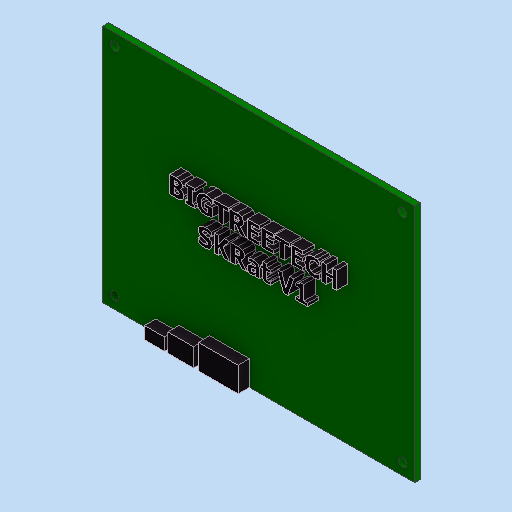
# Autodesk Inventor part: Bigtreetech Skrat V1
Saved by Autodesk Inventor 2023.2 (Build 272271000, 271)
## iProperties
Created: 2024-02-13
Part Number: Bigtreetech Skrat V1
Material: Generisch
Document SubType Name: Modeling
Designer: Nils Bade
Density: 1 g/cm^3
Appearance: Vorgabe
Auf Bestellliste: True
Author: Nils Bade
Autodesk Inventor part; units mm, degrees
ref_plane "YZ Plane" through (0, 0, 0) normal (1, 0, 0) x (0, 1, 0)
ref_plane "XZ Plane" through (0, 0, 0) normal (0, 1, 0) x (-1, 0, 0)
ref_plane "XY Plane" through (0, 0, 0) normal (0, 0, 1) x (1, 0, 0)
sketch "Skizze1" plane through (0, 0, 0) normal (0, 0, 1) x (1, 0, 0)
  line L0 (0, 0) -> (109.67, 0)
  line L1 (109.67, 0) -> (109.67, 84.3)
  line L2 (109.67, 84.3) -> (0, 84.3)
  line L3 (0, 84.3) -> (0, 0)
  circle A0 centre (3.98, 4) radius 1.5
  circle A1 centre (3.98, 80.1) radius 1.5
  circle A2 centre (105.33, 4) radius 1.5
  circle A3 centre (105.33, 80.1) radius 1.5
  line L4 (18.6, 0) -> (25.6, 0)
  line L5 (25.6, 0) -> (25.6, 4.3544)
  line L6 (25.6, 4.3544) -> (18.6, 4.3544)
  line L7 (18.6, 4.3544) -> (18.6, 0)
  line L8 (26.81, 0) -> (35.81, 0)
  line L9 (35.81, 0) -> (35.81, 6.5)
  line L10 (35.81, 6.5) -> (26.81, 6.5)
  line L11 (26.81, 6.5) -> (26.81, 0)
  line L12 (51.54, 0) -> (37.54, 0)
  line L13 (37.54, 0) -> (37.54, 8.7146)
  line L14 (37.54, 8.7146) -> (51.54, 8.7146)
  line L15 (51.54, 8.7146) -> (51.54, 0)
  line L16 (14.8977, 55.016) -> (98.7322, 55.016) construction
  line L17 (98.7322, 55.016) -> (98.7322, 43.3287) construction
  line L18 (98.7322, 43.3287) -> (14.8977, 43.3287) construction
  line L19 (14.8977, 43.3287) -> (14.8977, 55.016) construction
  circle A4 centre (3.98, 4) radius 3.5
  circle A5 centre (3.98, 80.1) radius 3.5
  circle A6 centre (105.33, 80.1) radius 3.5
  circle A7 centre (105.33, 4) radius 3.5
  spline S0 degree 2 poles (32.3655, 50.6659) (32.3655, 50.2112) (32.0194, 49.524) (31.7327, 49.2966) knots 0 0 0 1 2 2 2
  spline S1 degree 2 poles (31.7327, 49.2966) (31.3867, 49.0248) (30.5661, 48.7974) (29.9284, 48.7974) knots 0 0 0 1 2 2 2
  line L20 (29.9284, 48.7974) -> (27.4914, 48.7974)
  line L21 (27.4914, 48.7974) -> (27.4914, 54.8974)
  line L22 (27.4914, 54.8974) -> (29.6417, 54.8974)
  spline S2 degree 2 poles (29.6417, 54.8974) (30.314, 54.8974) (31.0061, 54.7936) (31.3076, 54.6304) knots 0 0 0 1 2 2 2
  spline S3 degree 2 poles (31.3076, 54.6304) (31.6388, 54.4574) (31.9601, 53.8642) (31.9601, 53.4787) knots 0 0 0 1 2 2 2
  spline S4 degree 2 poles (31.9601, 53.4787) (31.9601, 53.0338) (31.5152, 52.3368) (31.1198, 52.1736) knots 0 0 0 1 2 2 2
  line L23 (31.1198, 52.1736) -> (31.1198, 52.144)
  spline S5 degree 2 poles (31.1198, 52.144) (31.6882, 52.0253) (32.3655, 51.2888) (32.3655, 50.6659) knots 0 0 0 1 2 2 2
  spline S6 degree 2 poles (30.7836, 50.6907) (30.7836, 50.9774) (30.5562, 51.2987) (30.3288, 51.3827) knots 0 0 0 1 2 2 2
  spline S7 degree 2 poles (30.3288, 51.3827) (30.1904, 51.4371) (29.701, 51.447) (29.2957, 51.447) knots 0 0 0 1 2 2 2
  line L24 (29.2957, 51.447) -> (29.0139, 51.447)
  line L25 (29.0139, 51.447) -> (29.0139, 49.9096)
  line L26 (29.0139, 49.9096) -> (29.098, 49.9096)
  spline S8 degree 2 poles (29.098, 49.9096) (29.6912, 49.9096) (30.1459, 49.9244) (30.3832, 50.0283) knots 0 0 0 1 2 2 2
  spline S9 degree 2 poles (30.3832, 50.0283) (30.5908, 50.1222) (30.7836, 50.4682) (30.7836, 50.6907) knots 0 0 0 1 2 2 2
  spline S10 degree 2 poles (30.403, 53.1771) (30.403, 53.3254) (30.2498, 53.6368) (30.0916, 53.7061) knots 0 0 0 1 2 2 2
  spline S11 degree 2 poles (30.0916, 53.7061) (29.9433, 53.7753) (29.528, 53.7851) (29.1177, 53.7851) knots 0 0 0 1 2 2 2
  line L27 (29.1177, 53.7851) -> (29.0139, 53.7851)
  line L28 (29.0139, 53.7851) -> (29.0139, 52.49)
  line L29 (29.0139, 52.49) -> (29.2067, 52.49)
  spline S12 degree 2 poles (29.2067, 52.49) (29.5972, 52.49) (29.9136, 52.5048) (30.0817, 52.5839) knots 0 0 0 1 2 2 2
  spline S13 degree 2 poles (30.0817, 52.5839) (30.2646, 52.6729) (30.403, 52.9744) (30.403, 53.1771) knots 0 0 0 1 2 2 2
  line L30 (36.2805, 48.7974) -> (32.9982, 48.7974)
  line L31 (32.9982, 48.7974) -> (32.9982, 49.8602)
  line L32 (32.9982, 49.8602) -> (33.8732, 49.8602)
  line L33 (33.8732, 49.8602) -> (33.8732, 53.8346)
  line L34 (33.8732, 53.8346) -> (32.9982, 53.8346)
  line L35 (32.9982, 53.8346) -> (32.9982, 54.8974)
  line L36 (32.9982, 54.8974) -> (36.2805, 54.8974)
  line L37 (36.2805, 54.8974) -> (36.2805, 53.8346)
  line L38 (36.2805, 53.8346) -> (35.4056, 53.8346)
  line L39 (35.4056, 53.8346) -> (35.4056, 49.8602)
  line L40 (35.4056, 49.8602) -> (36.2805, 49.8602)
  line L41 (36.2805, 49.8602) -> (36.2805, 48.7974)
  spline S14 degree 2 poles (42.3904, 49.1434) (41.99, 48.9803) (40.7097, 48.6689) (40.0869, 48.6689) knots 0 0 0 1 2 2 2
  spline S15 degree 2 poles (40.0869, 48.6689) (38.6484, 48.6689) (36.9429, 50.3298) (36.9429, 51.8523) knots 0 0 0 1 2 2 2
  spline S16 degree 2 poles (36.9429, 51.8523) (36.9429, 53.2859) (38.6484, 55.016) (40.1314, 55.016) knots 0 0 0 1 2 2 2
  spline S17 degree 2 poles (40.1314, 55.016) (40.8976, 55.016) (41.8566, 54.7244) (42.3657, 54.4772) knots 0 0 0 1 2 2 2
  line L42 (42.3657, 54.4772) -> (42.3657, 53.0437)
  line L43 (42.3657, 53.0437) -> (42.2273, 53.0437)
  spline S18 degree 2 poles (42.2273, 53.0437) (42.1186, 53.1277) (41.7033, 53.449) (41.5056, 53.5578) knots 0 0 0 1 2 2 2
  spline S19 degree 2 poles (41.5056, 53.5578) (41.2782, 53.6912) (40.6751, 53.8791) (40.339, 53.8791) knots 0 0 0 1 2 2 2
  spline S20 degree 2 poles (40.339, 53.8791) (39.9485, 53.8791) (39.3009, 53.6319) (39.0488, 53.3798) knots 0 0 0 1 2 2 2
  spline S21 degree 2 poles (39.0488, 53.3798) (38.8066, 53.1326) (38.5248, 52.3763) (38.5248, 51.877) knots 0 0 0 1 2 2 2
  spline S22 degree 2 poles (38.5248, 51.877) (38.5248, 50.8093) (39.5975, 49.791) (40.5219, 49.791) knots 0 0 0 1 2 2 2
  spline S23 degree 2 poles (40.5219, 49.791) (40.6059, 49.791) (40.8234, 49.8009) (40.9075, 49.8058) knots 0 0 0 1 2 2 2
  line L44 (40.9075, 49.8058) -> (40.9075, 51.007)
  line L45 (40.9075, 51.007) -> (39.726, 51.007)
  line L46 (39.726, 51.007) -> (39.726, 52.1489)
  line L47 (39.726, 52.1489) -> (42.3904, 52.1489)
  line L48 (42.3904, 52.1489) -> (42.3904, 49.1434)
  line L49 (44.7187, 48.7974) -> (44.7187, 53.7357)
  line L50 (44.7187, 53.7357) -> (42.9144, 53.7357)
  line L51 (42.9144, 53.7357) -> (42.9144, 54.8974)
  line L52 (42.9144, 54.8974) -> (48.0554, 54.8974)
  line L53 (48.0554, 54.8974) -> (48.0554, 53.7357)
  line L54 (48.0554, 53.7357) -> (46.2511, 53.7357)
  line L55 (46.2511, 53.7357) -> (46.2511, 48.7974)
  line L56 (46.2511, 48.7974) -> (44.7187, 48.7974)
  line L57 (54.3186, 48.7974) -> (52.4549, 48.7974)
  line L58 (52.4549, 48.7974) -> (50.7594, 51.0367)
  line L59 (50.7594, 51.0367) -> (50.2058, 51.0367)
  line L60 (50.2058, 51.0367) -> (50.2058, 48.7974)
  line L61 (50.2058, 48.7974) -> (48.6832, 48.7974)
  line L62 (48.6832, 48.7974) -> (48.6832, 54.8974)
  line L63 (48.6832, 54.8974) -> (51.1351, 54.8974)
  spline S24 degree 2 poles (51.1351, 54.8974) (51.6442, 54.8974) (52.3956, 54.7689) (52.7169, 54.5711) knots 0 0 0 1 2 2 2
  spline S25 degree 2 poles (52.7169, 54.5711) (53.0432, 54.3635) (53.4288, 53.7159) (53.4288, 53.2216) knots 0 0 0 1 2 2 2
  spline S26 degree 2 poles (53.4288, 53.2216) (53.4288, 52.5246) (52.796, 51.6496) (52.2671, 51.3926) knots 0 0 0 1 2 2 2
  line L64 (52.2671, 51.3926) -> (54.3186, 48.7974)
  spline S27 degree 2 poles (51.8568, 53.0288) (51.8568, 53.2612) (51.6788, 53.5924) (51.4762, 53.6813) knots 0 0 0 1 2 2 2
  spline S28 degree 2 poles (51.4762, 53.6813) (51.3328, 53.7407) (50.9818, 53.7753) (50.7199, 53.7753) knots 0 0 0 1 2 2 2
  line L65 (50.7199, 53.7753) -> (50.2058, 53.7753)
  line L66 (50.2058, 53.7753) -> (50.2058, 52.1341)
  line L67 (50.2058, 52.1341) -> (50.6457, 52.1341)
  spline S29 degree 2 poles (50.6457, 52.1341) (50.9621, 52.1341) (51.4119, 52.2132) (51.5652, 52.3368) knots 0 0 0 1 2 2 2
  spline S30 degree 2 poles (51.5652, 52.3368) (51.7134, 52.4554) (51.8568, 52.7718) (51.8568, 53.0288) knots 0 0 0 1 2 2 2
  line L68 (54.7733, 48.7974) -> (54.7733, 54.8974)
  line L69 (54.7733, 54.8974) -> (58.896, 54.8974)
  line L70 (58.896, 54.8974) -> (58.896, 53.7357)
  line L71 (58.896, 53.7357) -> (56.2959, 53.7357)
  line L72 (56.2959, 53.7357) -> (56.2959, 52.663)
  line L73 (56.2959, 52.663) -> (58.6934, 52.663)
  line L74 (58.6934, 52.663) -> (58.6934, 51.5014)
  line L75 (58.6934, 51.5014) -> (56.2959, 51.5014)
  line L76 (56.2959, 51.5014) -> (56.2959, 49.959)
  line L77 (56.2959, 49.959) -> (58.896, 49.959)
  line L78 (58.896, 49.959) -> (58.896, 48.7974)
  line L79 (58.896, 48.7974) -> (54.7733, 48.7974)
  line L80 (59.9341, 48.7974) -> (59.9341, 54.8974)
  line L81 (59.9341, 54.8974) -> (64.0568, 54.8974)
  line L82 (64.0568, 54.8974) -> (64.0568, 53.7357)
  line L83 (64.0568, 53.7357) -> (61.4566, 53.7357)
  line L84 (61.4566, 53.7357) -> (61.4566, 52.663)
  line L85 (61.4566, 52.663) -> (63.8541, 52.663)
  line L86 (63.8541, 52.663) -> (63.8541, 51.5014)
  line L87 (63.8541, 51.5014) -> (61.4566, 51.5014)
  line L88 (61.4566, 51.5014) -> (61.4566, 49.959)
  line L89 (61.4566, 49.959) -> (64.0568, 49.959)
  line L90 (64.0568, 49.959) -> (64.0568, 48.7974)
  line L91 (64.0568, 48.7974) -> (59.9341, 48.7974)
  line L92 (66.2664, 48.7974) -> (66.2664, 53.7357)
  line L93 (66.2664, 53.7357) -> (64.4622, 53.7357)
  line L94 (64.4622, 53.7357) -> (64.4622, 54.8974)
  line L95 (64.4622, 54.8974) -> (69.6032, 54.8974)
  line L96 (69.6032, 54.8974) -> (69.6032, 53.7357)
  line L97 (69.6032, 53.7357) -> (67.7989, 53.7357)
  line L98 (67.7989, 53.7357) -> (67.7989, 48.7974)
  line L99 (67.7989, 48.7974) -> (66.2664, 48.7974)
  line L100 (70.231, 48.7974) -> (70.231, 54.8974)
  line L101 (70.231, 54.8974) -> (74.3536, 54.8974)
  line L102 (74.3536, 54.8974) -> (74.3536, 53.7357)
  line L103 (74.3536, 53.7357) -> (71.7535, 53.7357)
  line L104 (71.7535, 53.7357) -> (71.7535, 52.663)
  line L105 (71.7535, 52.663) -> (74.151, 52.663)
  line L106 (74.151, 52.663) -> (74.151, 51.5014)
  line L107 (74.151, 51.5014) -> (71.7535, 51.5014)
  line L108 (71.7535, 51.5014) -> (71.7535, 49.959)
  line L109 (71.7535, 49.959) -> (74.3536, 49.959)
  line L110 (74.3536, 49.959) -> (74.3536, 48.7974)
  line L111 (74.3536, 48.7974) -> (70.231, 48.7974)
  spline S31 degree 2 poles (78.0216, 48.6787) (76.6473, 48.6787) (75.0358, 50.3397) (75.0358, 51.8424) knots 0 0 0 1 2 2 2
  spline S32 degree 2 poles (75.0358, 51.8424) (75.0358, 53.2908) (76.6523, 55.016) (78.0265, 55.016) knots 0 0 0 1 2 2 2
  spline S33 degree 2 poles (78.0265, 55.016) (78.3874, 55.016) (78.9707, 54.932) (79.2376, 54.8628) knots 0 0 0 1 2 2 2
  spline S34 degree 2 poles (79.2376, 54.8628) (79.4452, 54.7985) (79.9346, 54.586) (80.0878, 54.5069) knots 0 0 0 1 2 2 2
  line L112 (80.0878, 54.5069) -> (80.0878, 53.0535)
  line L113 (80.0878, 53.0535) -> (79.9346, 53.0535)
  spline S35 degree 2 poles (79.9346, 53.0535) (79.8209, 53.1524) (79.4848, 53.4292) (79.2722, 53.5578) knots 0 0 0 1 2 2 2
  spline S36 degree 2 poles (79.2722, 53.5578) (79.0596, 53.6912) (78.5505, 53.8741) (78.2687, 53.8741) knots 0 0 0 1 2 2 2
  spline S37 degree 2 poles (78.2687, 53.8741) (77.9375, 53.8741) (77.3888, 53.6665) (77.1367, 53.4045) knots 0 0 0 1 2 2 2
  spline S38 degree 2 poles (77.1367, 53.4045) (76.9093, 53.1722) (76.6177, 52.3763) (76.6177, 51.8375) knots 0 0 0 1 2 2 2
  spline S39 degree 2 poles (76.6177, 51.8375) (76.6177, 51.269) (76.9192, 50.4929) (77.1664, 50.2556) knots 0 0 0 1 2 2 2
  spline S40 degree 2 poles (77.1664, 50.2556) (77.4036, 50.0233) (77.987, 49.8206) (78.2786, 49.8206) knots 0 0 0 1 2 2 2
  spline S41 degree 2 poles (78.2786, 49.8206) (78.5801, 49.8206) (79.1288, 50.0233) (79.3167, 50.1469) knots 0 0 0 1 2 2 2
  spline S42 degree 2 poles (79.3167, 50.1469) (79.5243, 50.2705) (79.8357, 50.5325) (79.9494, 50.6363) knots 0 0 0 1 2 2 2
  line L114 (79.9494, 50.6363) -> (80.0878, 50.6363)
  line L115 (80.0878, 50.6363) -> (80.0878, 49.2027)
  spline S43 degree 2 poles (80.0878, 49.2027) (79.9198, 49.1236) (79.4798, 48.9259) (79.2425, 48.8567) knots 0 0 0 1 2 2 2
  spline S44 degree 2 poles (79.2425, 48.8567) (78.9558, 48.7677) (78.4566, 48.6787) (78.0216, 48.6787) knots 0 0 0 1 2 2 2
  line L116 (86.1384, 48.7974) -> (84.606, 48.7974)
  line L117 (84.606, 48.7974) -> (84.606, 51.5014)
  line L118 (84.606, 51.5014) -> (82.5249, 51.5014)
  line L119 (82.5249, 51.5014) -> (82.5249, 48.7974)
  line L120 (82.5249, 48.7974) -> (80.9925, 48.7974)
  line L121 (80.9925, 48.7974) -> (80.9925, 54.8974)
  line L122 (80.9925, 54.8974) -> (82.5249, 54.8974)
  line L123 (82.5249, 54.8974) -> (82.5249, 52.663)
  line L124 (82.5249, 52.663) -> (84.606, 52.663)
  line L125 (84.606, 52.663) -> (84.606, 54.8974)
  line L126 (84.606, 54.8974) -> (86.1384, 54.8974)
  line L127 (86.1384, 54.8974) -> (86.1384, 48.7974)
  spline S45 degree 2 poles (39.7235, 38.6451) (39.0216, 38.6451) (37.9637, 38.917) (37.509, 39.1147) knots 0 0 0 1 2 2 2
  line L128 (37.509, 39.1147) -> (37.509, 40.5681)
  line L129 (37.509, 40.5681) -> (37.6474, 40.5681)
  spline S46 degree 2 poles (37.6474, 40.5681) (38.1071, 40.1776) (39.2094, 39.7574) (39.7285, 39.7574) knots 0 0 0 1 2 2 2
  spline S47 degree 2 poles (39.7285, 39.7574) (39.8619, 39.7574) (40.292, 39.8167) (40.4205, 39.876) knots 0 0 0 1 2 2 2
  spline S48 degree 2 poles (40.4205, 39.876) (40.5787, 39.9452) (40.8012, 40.1973) (40.8012, 40.4) knots 0 0 0 1 2 2 2
  spline S49 degree 2 poles (40.8012, 40.4) (40.8012, 40.6323) (40.4403, 40.919) (40.1931, 40.9833) knots 0 0 0 1 2 2 2
  spline S50 degree 2 poles (40.1931, 40.9833) (39.8817, 41.0673) (39.1748, 41.2107) (38.8634, 41.3194) knots 0 0 0 1 2 2 2
  spline S51 degree 2 poles (38.8634, 41.3194) (38.1565, 41.5666) (37.5436, 42.4119) (37.5436, 43.0447) knots 0 0 0 1 2 2 2
  spline S52 degree 2 poles (37.5436, 43.0447) (37.5436, 43.8998) (38.9919, 44.9626) (40.0795, 44.9626) knots 0 0 0 1 2 2 2
  spline S53 degree 2 poles (40.0795, 44.9626) (40.6232, 44.9626) (41.7008, 44.7402) (42.126, 44.5523) knots 0 0 0 1 2 2 2
  line L130 (42.126, 44.5523) -> (42.126, 43.1583)
  line L131 (42.126, 43.1583) -> (41.9925, 43.1583)
  spline S54 degree 2 poles (41.9925, 43.1583) (41.6514, 43.45) (40.6726, 43.8504) (40.1585, 43.8504) knots 0 0 0 1 2 2 2
  spline S55 degree 2 poles (40.1585, 43.8504) (39.9559, 43.8504) (39.6395, 43.7911) (39.4615, 43.712) knots 0 0 0 1 2 2 2
  spline S56 degree 2 poles (39.4615, 43.712) (39.3182, 43.6477) (39.1106, 43.3907) (39.1106, 43.2325) knots 0 0 0 1 2 2 2
  spline S57 degree 2 poles (39.1106, 43.2325) (39.1106, 42.9952) (39.4418, 42.7233) (39.9163, 42.6146) knots 0 0 0 1 2 2 2
  spline S58 degree 2 poles (39.9163, 42.6146) (40.2228, 42.5454) (40.7913, 42.4119) (41.1175, 42.2982) knots 0 0 0 1 2 2 2
  spline S59 degree 2 poles (41.1175, 42.2982) (41.7503, 42.0659) (42.3682, 41.2947) (42.3682, 40.662) knots 0 0 0 1 2 2 2
  spline S60 degree 2 poles (42.3682, 40.662) (42.3682, 39.7524) (40.9396, 38.6451) (39.7235, 38.6451) knots 0 0 0 1 2 2 2
  line L132 (48.4978, 38.7539) -> (46.6441, 38.7539)
  line L133 (46.6441, 38.7539) -> (44.9881, 41.2305)
  line L134 (44.9881, 41.2305) -> (44.6866, 40.8152)
  line L135 (44.6866, 40.8152) -> (44.6866, 38.7539)
  line L136 (44.6866, 38.7539) -> (43.1542, 38.7539)
  line L137 (43.1542, 38.7539) -> (43.1542, 44.8539)
  line L138 (43.1542, 44.8539) -> (44.6866, 44.8539)
  line L139 (44.6866, 44.8539) -> (44.6866, 42.1301)
  line L140 (44.6866, 42.1301) -> (46.6441, 44.8539)
  line L141 (46.6441, 44.8539) -> (48.4089, 44.8539)
  line L142 (48.4089, 44.8539) -> (46.2338, 42.0214)
  line L143 (46.2338, 42.0214) -> (48.4978, 38.7539)
  line L144 (54.6325, 38.7539) -> (52.7688, 38.7539)
  line L145 (52.7688, 38.7539) -> (51.0733, 40.9932)
  line L146 (51.0733, 40.9932) -> (50.5196, 40.9932)
  line L147 (50.5196, 40.9932) -> (50.5196, 38.7539)
  line L148 (50.5196, 38.7539) -> (48.9971, 38.7539)
  line L149 (48.9971, 38.7539) -> (48.9971, 44.8539)
  line L150 (48.9971, 44.8539) -> (51.449, 44.8539)
  spline S61 degree 2 poles (51.449, 44.8539) (51.9581, 44.8539) (52.7095, 44.7254) (53.0308, 44.5276) knots 0 0 0 1 2 2 2
  spline S62 degree 2 poles (53.0308, 44.5276) (53.3571, 44.32) (53.7427, 43.6724) (53.7427, 43.1781) knots 0 0 0 1 2 2 2
  spline S63 degree 2 poles (53.7427, 43.1781) (53.7427, 42.4811) (53.1099, 41.6062) (52.581, 41.3491) knots 0 0 0 1 2 2 2
  line L151 (52.581, 41.3491) -> (54.6325, 38.7539)
  spline S64 degree 2 poles (52.1707, 42.9853) (52.1707, 43.2177) (51.9927, 43.5489) (51.7901, 43.6378) knots 0 0 0 1 2 2 2
  spline S65 degree 2 poles (51.7901, 43.6378) (51.6467, 43.6972) (51.2957, 43.7318) (51.0337, 43.7318) knots 0 0 0 1 2 2 2
  line L152 (51.0337, 43.7318) -> (50.5196, 43.7318)
  line L153 (50.5196, 43.7318) -> (50.5196, 42.0906)
  line L154 (50.5196, 42.0906) -> (50.9596, 42.0906)
  spline S66 degree 2 poles (50.9596, 42.0906) (51.276, 42.0906) (51.7258, 42.1697) (51.879, 42.2933) knots 0 0 0 1 2 2 2
  spline S67 degree 2 poles (51.879, 42.2933) (52.0273, 42.4119) (52.1707, 42.7283) (52.1707, 42.9853) knots 0 0 0 1 2 2 2
  spline S68 degree 2 poles (57.5391, 39.2433) (57.3908, 39.1197) (57.1585, 38.922) (56.9607, 38.8231) knots 0 0 0 1 2 2 2
  spline S69 degree 2 poles (56.9607, 38.8231) (56.7679, 38.7292) (56.4021, 38.6303) (56.0759, 38.6303) knots 0 0 0 1 2 2 2
  spline S70 degree 2 poles (56.0759, 38.6303) (55.4629, 38.6303) (54.6572, 39.4509) (54.6572, 40.0737) knots 0 0 0 1 2 2 2
  spline S71 degree 2 poles (54.6572, 40.0737) (54.6572, 40.5829) (55.0675, 41.2156) (55.453, 41.3985) knots 0 0 0 1 2 2 2
  spline S72 degree 2 poles (55.453, 41.3985) (55.8436, 41.5864) (56.9261, 41.7347) (57.549, 41.7742) knots 0 0 0 1 2 2 2
  line L155 (57.549, 41.7742) -> (57.549, 41.7989)
  spline S73 degree 2 poles (57.549, 41.7989) (57.549, 42.1796) (56.9855, 42.4712) (56.4219, 42.4712) knots 0 0 0 1 2 2 2
  spline S74 degree 2 poles (56.4219, 42.4712) (56.1698, 42.4712) (55.4876, 42.2883) (55.1663, 42.145) knots 0 0 0 1 2 2 2
  line L156 (55.1663, 42.145) -> (55.0427, 42.145)
  line L157 (55.0427, 42.145) -> (55.0427, 43.2572)
  spline S75 degree 2 poles (55.0427, 43.2572) (55.2553, 43.3165) (56.2044, 43.4846) (56.6889, 43.4846) knots 0 0 0 1 2 2 2
  spline S76 degree 2 poles (56.6889, 43.4846) (57.8752, 43.4846) (58.9628, 42.6937) (58.9628, 41.883) knots 0 0 0 1 2 2 2
  line L158 (58.9628, 41.883) -> (58.9628, 38.7539)
  line L159 (58.9628, 38.7539) -> (57.5391, 38.7539)
  line L160 (57.5391, 38.7539) -> (57.5391, 39.2433)
  line L161 (57.5391, 39.9551) -> (57.5391, 40.9092)
  spline S77 degree 2 poles (57.5391, 40.9092) (57.1733, 40.8746) (56.7235, 40.8202) (56.506, 40.7411) knots 0 0 0 1 2 2 2
  spline S78 degree 2 poles (56.506, 40.7411) (56.3132, 40.6768) (56.1055, 40.4099) (56.1055, 40.1924) knots 0 0 0 1 2 2 2
  spline S79 degree 2 poles (56.1055, 40.1924) (56.1055, 39.8711) (56.4565, 39.6288) (56.7976, 39.6288) knots 0 0 0 1 2 2 2
  spline S80 degree 2 poles (56.7976, 39.6288) (56.9855, 39.6288) (57.3809, 39.8019) (57.5391, 39.9551) knots 0 0 0 1 2 2 2
  spline S81 degree 2 poles (61.7854, 38.6649) (60.9104, 38.6649) (60.1096, 39.3866) (60.1096, 40.2072) knots 0 0 0 1 2 2 2
  line L162 (60.1096, 40.2072) -> (60.1096, 42.3575)
  line L163 (60.1096, 42.3575) -> (59.5609, 42.3575)
  line L164 (59.5609, 42.3575) -> (59.5609, 43.3561)
  line L165 (59.5609, 43.3561) -> (60.1096, 43.3561)
  line L166 (60.1096, 43.3561) -> (60.1096, 44.671)
  line L167 (60.1096, 44.671) -> (61.5431, 44.671)
  line L168 (61.5431, 44.671) -> (61.5431, 43.3561)
  line L169 (61.5431, 43.3561) -> (62.9273, 43.3561)
  line L170 (62.9273, 43.3561) -> (62.9273, 42.3575)
  line L171 (62.9273, 42.3575) -> (61.5431, 42.3575)
  line L172 (61.5431, 42.3575) -> (61.5431, 40.7213)
  spline S82 degree 2 poles (61.5431, 40.7213) (61.5431, 40.4791) (61.553, 40.1182) (61.6124, 39.9749) knots 0 0 0 1 2 2 2
  spline S83 degree 2 poles (61.6124, 39.9749) (61.6717, 39.8315) (61.9633, 39.6635) (62.2402, 39.6635) knots 0 0 0 1 2 2 2
  spline S84 degree 2 poles (62.2402, 39.6635) (62.3588, 39.6635) (62.7295, 39.7623) (62.8037, 39.8019) knots 0 0 0 1 2 2 2
  line L173 (62.8037, 39.8019) -> (62.9273, 39.8019)
  line L174 (62.9273, 39.8019) -> (62.9273, 38.7934)
  spline S85 degree 2 poles (62.9273, 38.7934) (62.6949, 38.7341) (62.1709, 38.6649) (61.7854, 38.6649) knots 0 0 0 1 2 2 2
  line L175 (71.143, 44.8539) -> (69.047, 38.7539)
  line L176 (69.047, 38.7539) -> (67.4504, 38.7539)
  line L177 (67.4504, 38.7539) -> (65.3544, 44.8539)
  line L178 (65.3544, 44.8539) -> (66.9412, 44.8539)
  line L179 (66.9412, 44.8539) -> (68.2709, 40.7164)
  line L180 (68.2709, 40.7164) -> (69.5957, 44.8539)
  line L181 (69.5957, 44.8539) -> (71.143, 44.8539)
  line L182 (75.9083, 38.7539) -> (71.8795, 38.7539)
  line L183 (71.8795, 38.7539) -> (71.8795, 39.8167)
  line L184 (71.8795, 39.8167) -> (73.1648, 39.8167)
  line L185 (73.1648, 39.8167) -> (73.1648, 43.0447)
  line L186 (73.1648, 43.0447) -> (71.8795, 43.0447)
  line L187 (71.8795, 43.0447) -> (71.8795, 44.0382)
  spline S86 degree 2 poles (71.8795, 44.0382) (72.1613, 44.0382) (72.7199, 44.1124) (72.888, 44.1915) knots 0 0 0 1 2 2 2
  spline S87 degree 2 poles (72.888, 44.1915) (73.0808, 44.2904) (73.2983, 44.6216) (73.318, 44.8687) knots 0 0 0 1 2 2 2
  line L188 (73.318, 44.8687) -> (74.6527, 44.8687)
  line L189 (74.6527, 44.8687) -> (74.6527, 39.8167)
  line L190 (74.6527, 39.8167) -> (75.9083, 39.8167)
  line L191 (75.9083, 39.8167) -> (75.9083, 38.7539)
  point P0 (22.1, 4.3544)
  point P1 (31.31, 6.5)
  point P2 (44.54, 8.7146)
  dimension "d0" = 109.67
  dimension "d1" = 84.3
  dimension "d2" = 3
  dimension "d3" = 3.98
  dimension "d4" = 4
  dimension "d7" = 76.1
  dimension "d14" = 101.35
  dimension "d19" = 22.1
  dimension "d20" = 31.31
  dimension "d21" = 44.54
  dimension "d22" = 7
  dimension "d23" = 9
  dimension "d24" = 14
  dimension "d29" = 7
  dimension "d30" = 7
  dimension "d31" = 7
  dimension "d32" = 7
  constraints: 32 end point, 8 centre point, 8 parallel, 5 horizontal, 4 coincident, 4 perpendicular, 3 midpoint, 3 point on line, 1 vertical, 8 other
  measures "d0" distance of L1.end L2.end
  measures "d1" distance of L2.end L0.start
  measures "d2" diameter of A0
  measures "d3" distance from line of L3 A0.centre
  measures "d4" distance from line of L0 A0.centre
  measures "d7" distance of A0.centre A1.centre
  measures "d14" distance of A0.centre A2.centre
  measures "d19" distance from line of L3 point (22.1, 4.354)
  measures "d20" distance from line of L3 point (31.31, 6.5)
  measures "d21" distance from line of L3 point (44.54, 8.715)
  measures "d22" distance of L5.end L6.end
  measures "d23" distance of L9.end L10.end
  measures "d24" distance of L13.end L14.end
  measures "d29" diameter of A4
  measures "d30" diameter of A5
  measures "d31" diameter of A6
  measures "d32" diameter of A7
extrude "Extrusion1" add sketch "Skizze1" along normal blind 2 contours L3 L2 L1 L0 L15 L14 L13 L9 L10 L11 L5 L6 L7 | L7 L6 L5 L0 | L11 L10 L9 L0 | L0 L13 L14 L15 | A4 | A5 | A6 | A7 | S0 S1 L20 L21 L22 S2 S3 S4 L23 S5 | S9 S8 L26 L25 L24 S7 S6 | S13 S12 L29 L28 L27 S11 S10 | L30 L31 L32 L33 L34 L35 L36 L37 L38 L39 L40 L41 | S14 S15 S16 S17 L42 L43 S18 S19 S20 S21 S22 S23 L44 L45 L46 L47 L48 | L49 L50 L51 L52 L53 L54 L55 L56 | L57 L58 L59 L60 L61 L62 L63 S24 S25 S26 L64 | S30 S29 L67 L66 L65 S28 S27 | L68 L69 L70 L71 L72 L73 L74 L75 L76 L77 L78 L79 | L80 L81 L82 L83 L84 L85 L86 L87 L88 L89 L90 L91 | L92 L93 L94 L95 L96 L97 L98 L99 | L100 L101 L102 L103 L104 L105 L106 L107 L108 L109 L110 L111 | S31 S32 S33 S34 L112 L113 S35 S36 S37 S38 S39 S40 S41 S42 L114 L115 S43 S44 | L116 L117 L118 L119 L120 L121 L122 L123 L124 L125 L126 L127 | S45 L128 L129 S46 S47 S48 S49 S50 S51 S52 S53 L130 L131 S54 S55 S56 S57 S58 S59 S60 | L132 L133 L134 L135 L136 L137 L138 L139 L140 L141 L142 L143 | L144 L145 L146 L147 L148 L149 L150 S61 S62 S63 L151 | S67 S66 L154 L153 L152 S65 S64 | S68 S69 S70 S71 S72 L155 S73 S74 L156 L157 S75 S76 L158 L159 L160 | S80 S79 S78 S77 L161 | S81 L162 L163 L164 L165 L166 L167 L168 L169 L170 L171 L172 S82 S83 S84 L173 L174 S85 | L175 L176 L177 L178 L179 L180 L181 | L182 L183 L184 L185 L186 L187 S86 S87 L188 L189 L190 L191
extrude "Extrusion2" add sketch "Skizze1" along normal blind 4 from surface at 2 separate body contours L7 L6 L5 L0 | L11 L10 L9 L0 | L0 L13 L14 L15 | S0 S1 L20 L21 L22 S2 S3 S4 L23 S5 | L30 L31 L32 L33 L34 L35 L36 L37 L38 L39 L40 L41 | S14 S15 S16 S17 L42 L43 S18 S19 S20 S21 S22 S23 L44 L45 L46 L47 L48 | L49 L50 L51 L52 L53 L54 L55 L56 | L57 L58 L59 L60 L61 L62 L63 S24 S25 S26 L64 | L68 L69 L70 L71 L72 L73 L74 L75 L76 L77 L78 L79 | L80 L81 L82 L83 L84 L85 L86 L87 L88 L89 L90 L91 | L92 L93 L94 L95 L96 L97 L98 L99 | L100 L101 L102 L103 L104 L105 L106 L107 L108 L109 L110 L111 | S31 S32 S33 S34 L112 L113 S35 S36 S37 S38 S39 S40 S41 S42 L114 L115 S43 S44 | L116 L117 L118 L119 L120 L121 L122 L123 L124 L125 L126 L127 | S45 L128 L129 S46 S47 S48 S49 S50 S51 S52 S53 L130 L131 S54 S55 S56 S57 S58 S59 S60 | L132 L133 L134 L135 L136 L137 L138 L139 L140 L141 L142 L143 | L144 L145 L146 L147 L148 L149 L150 S61 S62 S63 L151 | S68 S69 S70 S71 S72 L155 S73 S74 L156 L157 S75 S76 L158 L159 L160 | S81 L162 L163 L164 L165 L166 L167 L168 L169 L170 L171 L172 S82 S83 S84 L173 L174 S85 | L175 L176 L177 L178 L179 L180 L181 | L182 L183 L184 L185 L186 L187 S86 S87 L188 L189 L190 L191
extrude "Extrusion3" [suppressed]
